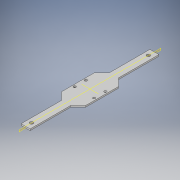
# Autodesk Inventor part: top beam
Saved by Autodesk Inventor 2017 (Build 210142000, 142)
## iProperties
Created: 2016-09-27
Part Number: top beam
Material: Generic
Document SubType Name: Modeling
Designer: Hanson
Density: 1 g/cm^3
Appearance: Default
Author: Hanson
Autodesk Inventor part; units mm, degrees
ref_plane "YZ Plane" through (0, 0, 0) normal (1, 0, 0) x (0, 1, 0)
ref_plane "XZ Plane" through (0, 0, 0) normal (0, 1, 0) x (-1, 0, 0)
ref_plane "XY Plane" through (0, 0, 0) normal (0, 0, 1) x (1, 0, 0)
sketch "Sketch1" plane through (0, 0, 0) normal (0, 1, 0) x (-1, 0, 0)
  line L0 (0, 0) -> (-19.05, 0)
  line L1 (-19.05, 0) -> (-19.05, -273.05)
  line L2 (-19.05, -273.05) -> (0, -273.05)
  line L3 (0, -273.05) -> (0, 0)
  dimension "d0" = 19.05
  dimension "d1" = 273.05
  constraints: 8 end point, 2 parallel, 1 horizontal, 1 perpendicular
  measures "d0" distance of L2.end L1.end
  measures "d1" distance of L1.end L0.end
extrude "Extrusion1" add sketch "Sketch1" along normal blind 3.175
sketch "Sketch2" plane through (0, 3.175, 0) normal (0, 1, 0) x (1, 0, 0)
  line L0 (0, 273.05) -> (0, 0) projected
  line L1 (0, 0) -> (19.05, 0) projected
  point P0 (9.525, 12.7)
  dimension "d4" = 9.525
  dimension "d5" = 12.7
  measures "d4" distance from line of L0 point (9.525, 12.7)
  measures "d5" distance from line of L1 point (9.525, 12.7)
hole "Hole1" at (9.525, 3.175, -12.7) direction (0, -1, 0) diameter 7.1374 end through all
sketch "Sketch4" plane through (19.05, 0, 0) normal (1, 0, 0) x (0, 0, -1)
  line L0 (273.05, 0) -> (273.05, 3.175) projected
  line L1 (0, 3.175) -> (273.05, 3.175)
  line L2 (273.05, 3.175) -> (273.05, 0)
  line L3 (273.05, 0) -> (0, 0)
  line L4 (0, 0) -> (0, 3.175)
  constraints: 8 end point, 2 parallel, 1 horizontal, 1 perpendicular
extrude "Extrusion2" add sketch "Sketch4" along normal blind 6.35
sketch "Sketch5" plane through (0, 0, -273.05) normal (-1, 0, 0) x (0, 0, 1)
  line L0 (0, 0) -> (0, 3.175) projected
  line L1 (0, 3.175) -> (273.05, 3.175)
  line L2 (273.05, 3.175) -> (273.05, 0)
  line L3 (273.05, 0) -> (0, 0)
  line L4 (0, 0) -> (0, 3.175)
  constraints: 8 end point, 2 parallel, 1 horizontal, 1 perpendicular
extrude "Extrusion3" add sketch "Sketch5" along normal blind 6.35
ref_plane "Work Plane1" through (9.525, 0, 0) normal (1, 0, 0) x (0, 0, -1)
ref_plane "Work Plane2" through (25.4, 0, -136.525) normal (0, 0, 1) x (1, 0, 0)
sketch "Sketch6" plane through (25.4, 0, 0) normal (1, 0, 0) x (0, 0, -1)
  line L0 (0, 0) -> (273.05, 0) projected
  line L1 (0, 3.175) -> (273.05, 3.175)
  line L2 (273.05, 3.175) -> (273.05, 0)
  line L3 (273.05, 0) -> (0, 0)
  line L4 (0, 0) -> (0, 3.175)
  constraints: 8 end point, 2 parallel, 1 horizontal, 1 perpendicular
extrude "Extrusion4" add sketch "Sketch6" along normal blind 9.525
sketch "Sketch7" plane through (-6.35, 0, -273.05) normal (-1, 0, 0) x (0, 0, 1)
  line L0 (273.05, 3.175) -> (0, 3.175) projected
  line L1 (0, 3.175) -> (0, 0) projected
  line L2 (273.05, 3.175) -> (0, 3.175)
  line L3 (0, 3.175) -> (0, 0)
  line L4 (0, 0) -> (273.05, 0)
  line L5 (273.05, 0) -> (273.05, 3.175)
  constraints: 8 end point, 2 parallel, 1 horizontal, 1 perpendicular
extrude "Extrusion5" add sketch "Sketch7" along normal blind 9.525
sketch "Sketch8" plane through (0, 3.175, 0) normal (0, 1, 0) x (1, 0, 0)
  line L0 (34.925, 273.05) -> (34.925, 0) projected
  line L1 (34.925, 0) -> (-15.875, 0) projected
  point P0 (0, 0)
  point P1 (30.1498, 124.6124)
  dimension "d30" = 4.7752
  dimension "d31" = 124.6124
  measures "d30" distance from line of L0 point (30.15, 124.612)
  measures "d31" distance from line of L1 point (30.15, 124.612)
hole "Hole3" at (30.1498, 3.175, -124.6124) direction (0, -1, 0) diameter 5.1816 end through all
mirror "Mirror4" about plane through (9.525, 0, 0) normal (1, 0, 0) of "Hole3"
mirror "Mirror5" about plane through (25.4, 0, -136.525) normal (0, 0, 1) of "Hole3", "Mirror4", "Hole1"
sketch "Sketch10" plane through (34.925, 0, 0) normal (1, 0, 0) x (0, 0, -1)
  line L0 (0, 3.175) -> (101.6, 3.175)
  line L1 (101.6, 3.175) -> (101.6, 0)
  line L2 (101.6, 0) -> (0, 0)
  line L3 (0, 0) -> (0, 3.175)
  dimension "d40" = 101.6
  dimension "d41" = 3.175
  constraints: 8 end point, 2 parallel, 1 horizontal, 1 perpendicular
  measures "d40" distance of L1.end L2.end
  measures "d41" distance of L0.end L1.end
extrude "Extrusion6" cut sketch "Sketch10" against normal blind 15.875
chamfer "Chamfer1" distance 15.875 angle 45 1 edges at (19.05, 1.5875, -101.6)
mirror "Mirror6" about plane through (9.525, 0, 0) normal (1, 0, 0) of "Extrusion6", "Chamfer1"
mirror "Mirror7" about plane through (25.4, 0, -136.525) normal (0, 0, 1) of "Extrusion6", "Chamfer1", "Mirror6"
body "Solid1"
